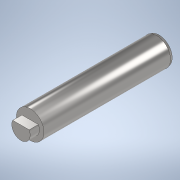
# Autodesk Inventor part: 平行ピンD6L30Dcut
Saved by Autodesk Inventor 2020.2 (Build 242310000, 310)
## iProperties
Created: 2020-02-29
Part Number: 平行ピンD6L30Dcut
Material: ステンレス鋼
Document SubType Name: Modeling
Designer: aoyam
Density: 8 g/cm^3
Appearance: 半つや出し
Author: aoyam
Autodesk Inventor part; units mm, degrees
ref_plane "YZ Plane" through (0, 0, 0) normal (1, 0, 0) x (0, 1, 0)
ref_plane "XZ Plane" through (0, 0, 0) normal (0, 1, 0) x (-1, 0, 0)
ref_plane "XY Plane" through (0, 0, 0) normal (0, 0, 1) x (1, 0, 0)
sketch "スケッチ1" plane through (0, 0, 0) normal (0, 0, 1) x (1, 0, 0)
  circle A0 centre (0, 0) radius 3
  dimension "d0" = 6
  constraints: 1 centre point, 1 coincident
  measures "d0" diameter of A0
extrude "押し出し1" add sketch "スケッチ1" along normal blind 30
chamfer "面取り1" distance 0.5 angle 15 2 edges at (-3, 0, 0) (-3, 0, 30) measured on face at (2.9903, -0.2414, 20)
sketch "スケッチ2" plane through (0, 0, 30) normal (0, 0, 1) x (1, 0, 0)
  circle A0 centre (0, 0) radius 3 projected
  circle A1 centre (0, 0) radius 2
  line L0 (-1.7861, 0.9) -> (1.7861, 0.9)
  dimension "d7" = 4
  dimension "d8" = 0.9
  constraints: 2 end point, 2 point on circle, 1 centre point, 1 coincident, 1 horizontal
  measures "d7" diameter of A1
  measures "d8" distance from line of point (0, 0) L0
extrude "押し出し2" cut sketch "スケッチ2" against normal blind 2 contours A0 | L0 A1 picked at (-0.2398, 1.4933)
